Autodesk Fusion 360 part; units mm, degrees
note: some values were not read from the file. Chosen so that the rebuilt part matches the saved one: a direction. Set by a fixed rule: which sketch regions a step uses.
(part 2 of 2)
component "BottomBox" placed x (1, 0, 0) y (0, 1, 0) z (0, 0, 1) at (0, 0, 0)
component "BackBox" placed x (1, 0, 0) y (0, 1, 0) z (0, 0, 1) at (0, 0, 0)
component "BoxSide" placed x (1, 0, 0) y (0, 1, 0) z (0, 0, 1) at (0, 0, 0)
component "BoxSeparator" placed x (1, 0, 0) y (0, 1, 0) z (0, 0, 1) at (0, 0, 0)
component "horizontaldowel" placed x (1, 0, 0) y (0, 1, 0) z (0, 0, 1) at (0, 0, 0)
component "camshaft" placed x (1, 0, 0) y (0, 1, 0) z (0, 0, 1) at (0, 0, 0)
component "dowel" placed x (1, 0, 0) y (0, 1, 0) z (0, 0, 1) at (0, 0, -29.4)
component "base" placed x (1, 0, 0) y (0, 1, 0) z (0, 0, 1) at (0, 0, -29.4)
component "mole" placed x (1, 0, 0) y (0, 1, 0) z (0, 0, 1) at (0, 0, 0)
component "BottomBox(Mirror)" placed x (1, 0, 0) y (0, 1, 0) z (0, 0, 1) at (0, 0, 153.4)
component "BoxSide(Mirror)" placed x (-1, 0, 0) y (0, 1, 0) z (0, 0, -1) at (0, 0, 0)
component "Shaft Holder" placed x (1, 0, 0) y (0, 1, 0) z (0, 0, 1) at (0, 0, 0)
component "dowel holder" placed x (1, 0, 0) y (0, 1, 0) z (0, 0, 1) at (0, 0, 0)
equation "width = 110 mm"
equation "length = 220 mm"
equation "height = 150 mm"
equation "num_fingers = 3"
equation "num_fingers_length = 6"
equation "thickness = 3.4 mm"
equation "d7 = length"
equation "d8 = width"
equation "d9 = length / ( num_fingers_length * 2 )"
equation "d10 = thickness"
equation "d11 = num_fingers_length"
equation "d13 = length / num_fingers_length"
equation "d15 = width / ( num_fingers * 2 )"
equation "d16 = thickness"
equation "d18 = num_fingers"
equation "d20 = width / num_fingers"
equation "d21 = thickness"
equation "d23 = length"
equation "d24 = height"
equation "d25 = height / ( num_fingers * 2 )"
equation "d26 = thickness"
equation "d28 = num_fingers"
equation "d30 = height / num_fingers"
equation "d31 = -thickness"
equation "d38 = height / 2 + thickness / 2"
equation "d39 = -thickness"
equation "d42 = width / 5"
equation "d43 = thickness"
equation "d44 = width / 5"
equation "d52 = length / 7"
equation "d53 = length / 7"
equation "d54 = thickness"
equation "d62 = height - 30 mm"
equation "d67 = length + ( thickness * 2 )"
equation "d68 = width"
equation "d69 = thickness"
equation "d70 = -thickness"
equation "d76 = length - ( length / 7 * 3 )"
equation "dowel_thickness = 4.8 mm"
equation "d80 = dowel_thickness"
equation "d81 = -thickness"
equation "d87 = -thickness"
equation "d89 = dowel_thickness"
equation "d90 = -length - ( thickness * 2 )"
equation "d92 = dowel_thickness"
equation "d95 = thickness / 2"
equation "d101 = thickness"
equation "d102 = length / ( num_fingers_length * 2 )"
equation "d103 = num_fingers_length"
equation "d105 = length / num_fingers_length"
equation "d107 = thickness / 2"
equation "d109 = dowel_thickness"
equation "d110 = -thickness"
equation "d113 = -thickness"
equation "d115 = dowel_thickness"
equation "d138 = length / 3"
equation "d142 = length / 3"
equation "d149 = thickness"
equation "d174 = thickness"
equation "d176 = dowel_thickness"
equation "d178 = thickness"
